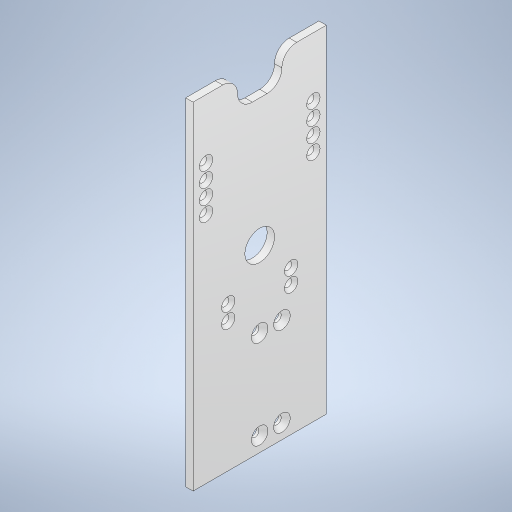
# Autodesk Inventor part: Bottom Plate
Saved by Autodesk Inventor 2023.4 (Build 274418000, 418)
## iProperties
Created: 2024-03-02
Part Number: Bottom Plate
Material: Aluminum 6061
Document SubType Name: Modeling
Designer: Nathan Cai
Mass: 67.3259 g
Surface Area: 177.704 cm^2
Volume: 24.9355 cm^3
Density: 2.7 g/cm^3
Appearance: Aluminum - Flat
Author: Nathan Cai
Autodesk Inventor part; units mm, degrees
ref_plane "YZ Plane" through (0, 0, 0) normal (1, 0, 0) x (0, 1, 0)
ref_plane "XZ Plane" through (0, 0, 0) normal (0, 1, 0) x (-1, 0, 0)
ref_plane "XY Plane" through (0, 0, 0) normal (0, 0, 1) x (1, 0, 0)
sketch "Sketch1" plane through (0, 0, 0) normal (1, 0, 0) x (0, 1, 0)
  line L0 (-73.8187, -28.575) -> (73.8188, -28.575)
  line L1 (73.8188, -28.575) -> (73.8187, 28.575)
  line L2 (73.8187, 28.575) -> (-73.8188, 28.575)
  line L3 (-73.8188, 28.575) -> (-73.8187, -28.575)
  line L4 (-73.8187, -28.575) -> (73.8187, 28.575) construction
  line L5 (73.8188, -28.575) -> (-73.8188, 28.575) construction
  line L6 (-73.8187, 0) -> (73.8188, 0) construction
  line L7 (86.5188, -9.525) -> (61.1188, -9.525)
  line L8 (61.1188, -9.525) -> (61.1188, 9.525)
  line L9 (61.1188, 9.525) -> (86.5188, 9.525)
  line L10 (86.5188, 9.525) -> (86.5188, -9.525)
  line L11 (86.5188, -9.525) -> (61.1188, 9.525) construction
  line L12 (61.1188, -9.525) -> (86.5188, 9.525) construction
  circle A0 centre (6.35, 0) radius 6.35
  line L13 (-73.8188, 28.575) -> (-70.6438, 28.575)
  line L14 (-70.6438, 28.575) -> (-70.6437, -28.575)
  line L15 (-70.6437, -28.575) -> (-73.8188, -28.575)
  line L16 (-73.8188, -28.575) -> (-73.8188, 28.575)
  point P0 (0, 0)
  point P1 (-24.6062, 0)
  point P2 (73.8187, -9.525)
  point P3 (73.8187, 9.525)
  point P4 (0, 0)
  point P5 (-70.6438, 28.575)
  dimension "d0" = 147.6375
  dimension "d1" = 57.15
  dimension "d36" = 25.4
  dimension "d37" = 19.05
  dimension "d46" = 12.7
  dimension "d48" = 6.35
  dimension "d49" = 3.175
  constraints: 34 end point, 7 midpoint, 6 parallel, 3 horizontal, 3 perpendicular, 3 point on line, 1 centre point
  measures "d0" distance of L2.end L1.end
  measures "d1" distance of L1.end L0.end
  measures "d36" distance of L8.end L9.end
  measures "d37" distance of L7.end L8.end
  measures "d46" diameter of A0
  measures "d48" distance of point (0, 0) A0.centre
  measures "d49" distance of L14.end L15.end
extrude "Extrusion1" add sketch "Sketch1" along normal blind 3.175 contours L14 L2 L1 L9 L8 L7 L0
fillet "Fillet2" radius 6.35 4 edges at (1.5875, 61.1188, 9.525) (1.5875, 73.8187, 9.525) (1.5875, 61.1188, -9.525) (1.5875, 73.8187, -9.525)
sketch "Sketch2" plane through (3.175, 0, 0) normal (1, 0, 0) x (0, 0, -1)
  point P0 (-23.0187, 48.4188)
  point P1 (-23.0187, 42.0688)
  point P2 (-23.0187, 35.7188)
  point P3 (-23.0187, 29.3688)
  point P4 (23.0188, 48.4188)
  point P5 (23.0188, 42.0688)
  point P6 (23.0188, 35.7188)
  point P7 (23.0188, 29.3688)
  point P8 (13.4938, -8.7312)
  point P9 (13.4938, -15.0812)
  point P10 (-13.4937, -8.7312)
  point P11 (-13.4937, -15.0812)
hole "Hole1" at (3.175, 48.4188, 23.0187) at (3.175, 42.0688, 23.0187) at (3.175, 35.7188, 23.0187) at (3.175, 29.3688, 23.0187) at (3.175, 48.4188, -23.0188) at (3.175, 42.0688, -23.0188) at (3.175, 35.7188, -23.0188) at (3.175, 29.3688, -23.0188) at (3.175, -8.7312, -13.4938) at (3.175, -15.0812, -13.4938) at (3.175, -8.7312, 13.4937) at (3.175, -15.0812, 13.4937) direction (-1, 0, 0) diameter 3.2639 end through all countersink diameter 5.715 countersink angle 82
sketch "Sketch3" plane through (3.175, 0, 0) normal (1, 0, 0) x (0, 0, -1)
  point P0 (0, -26.1937)
  point P1 (9.525, -26.1937)
  point P2 (9.525, -64.2937)
  point P3 (0, -64.2937)
hole "Hole2" at (3.175, -26.1937, 0) at (3.175, -26.1937, -9.525) at (3.175, -64.2937, -9.525) at (3.175, -64.2937, 0) direction (-1, 0, 0) diameter 3.5052 end through all countersink diameter 7.0866 countersink angle 82
body "Solid1"
